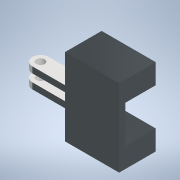
# Autodesk Inventor part: Tope_Carril
Saved by Autodesk Inventor 2022 (Build 260153000, 153)
## iProperties
Created: 2022-02-07
Part Number: Tope_Carril
Material: Generic
Document SubType Name: Modeling
Designer: katha
Density: 1 g/cm^3
Appearance: Default
Author: katha
Autodesk Inventor part; units mm, degrees
ref_plane "YZ Plane" through (0, 0, 0) normal (1, 0, 0) x (0, 1, 0)
ref_plane "XZ Plane" through (0, 0, 0) normal (0, 1, 0) x (-1, 0, 0)
ref_plane "XY Plane" through (0, 0, 0) normal (0, 0, 1) x (1, 0, 0)
sketch "Sketch1" plane through (0, 0, 0) normal (0, 0, 1) x (1, 0, 0)
  line L0 (0, 0) -> (20, 0) projected
  line L1 (20, 0) -> (20, 3.2) projected
  line L2 (0, 3.2) -> (20, 3.2) projected
  line L3 (0, 0) -> (0, 3.2) projected
  line L4 (20, -25) -> (0, -25) projected
  line L5 (0, -25) -> (0, -28.2) projected
  line L6 (20, -28.2) -> (0, -28.2) projected
  line L7 (20, -25) -> (20, -28.2) projected
  line L8 (3.2, -25) -> (3.2, 0) projected
  line L9 (0, -25) -> (0, 0) projected
  line L10 (-0.3, -0.3) -> (-0.3, 3.5)
  line L11 (-0.3, 3.5) -> (20.3, 3.5)
  line L12 (20.3, 3.5) -> (20.3, -0.3)
  line L13 (20.3, -24.7) -> (20.3, -28.5)
  line L14 (20.3, -28.5) -> (-0.3, -28.5)
  line L15 (-0.3, -28.5) -> (-0.3, -24.7)
  line L16 (3.5, -24.7) -> (3.5, -0.3)
  line L17 (-0.3, -0.3) -> (-0.3, -24.7)
  line L18 (20.3, -0.3) -> (3.5, -0.3)
  line L19 (3.5, -24.7) -> (20.3, -24.7)
  line L20 (6.5, -3.3) -> (6.5, -21.7)
  line L21 (6.5, -21.7) -> (23.3, -21.7)
  line L22 (23.3, -21.7) -> (23.3, -31.5)
  line L23 (23.3, -31.5) -> (-3.3, -31.5)
  line L24 (-3.3, -31.5) -> (-3.3, -24.7)
  line L25 (-3.3, -24.7) -> (-3.3, -0.3)
  line L26 (-3.3, -0.3) -> (-3.3, 6.5)
  line L27 (-3.3, 6.5) -> (23.3, 6.5)
  line L28 (23.3, 6.5) -> (23.3, -3.3)
  line L29 (23.3, -3.3) -> (6.5, -3.3)
  dimension "d2" = 0.3
  dimension "d3" = 0.3
  dimension "d4" = 0.3
  dimension "d5" = 24.4
  dimension "d6" = 3.8
  dimension "d7" = 3
  constraints: 40 end point, 3 equal length, 1 parallel, 13 other
  measures "d2" distance between parallel lines of L8 L16
  measures "d3" distance between parallel lines of L0 L18
  measures "d4" distance between parallel lines of L11 L2
  measures "d5" distance of L10.start L15.end
  measures "d6" distance of L10.start L10.end
  measures "d7" distance between parallel lines of L16 L20
extrude "Extrusion1" add sketch "Sketch1" against normal blind 15 contours L20 L21 L22 L23 L24 L25 L26 L27 L28 L29
sketch "Sketch4" plane through (0, 0, 0) normal (0, 0, 1) x (1, 0, 0)
  line L0 (23.3, -3.3) -> (23.3, 6.5) projected
  line L1 (23.3, 6.5) -> (-3.3, 6.5) projected
  line L2 (23.3, -3.3) -> (6.5, -3.3) projected
  line L3 (6.5, -3.3) -> (6.5, -21.7) projected
  line L4 (6.5, -21.7) -> (23.3, -21.7) projected
  line L5 (-3.3, -0.3) -> (-3.3, 6.5) projected
  line L6 (-3.3, -31.5) -> (23.3, -31.5) projected
  line L7 (23.3, -31.5) -> (23.3, -21.7) projected
  line L8 (23.3, -21.7) -> (6.5, -21.7) projected
  line L9 (23.3, 6.5) -> (23.3, -3.3) projected
  line L10 (23.3, -3.3) -> (23.3, 6.5)
  line L11 (-3.3, -31.5) -> (-3.3, 6.5) projected
  line L12 (23.3, 6.5) -> (-3.3, 6.5)
  line L13 (-3.3, 6.5) -> (-3.3, -31.5)
  line L14 (23.3, -31.5) -> (-3.3, -31.5) projected
  line L15 (-3.3, -31.5) -> (23.3, -31.5)
  line L16 (23.3, -21.7) -> (23.3, -31.5) projected
  line L17 (23.3, -31.5) -> (23.3, -21.7)
  line L18 (6.5, -3.3) -> (6.5, -21.7) projected
  line L19 (23.3, -3.3) -> (6.5, -3.3) projected
  line L20 (6.5, -3.3) -> (23.3, -3.3) projected
  line L21 (23.3, -3.3) -> (23.3, -21.7)
  point P0 (0, 0)
  constraints: 12 end point, 5 collinear, 1 perpendicular
extrude "Extrusion3" add sketch "Sketch4" along normal blind 3
sketch "Sketch5" plane through (6.5, -21.7, -15) normal (1, 0, 0) x (0, 0, -1)
  line L0 (0, 18.4) -> (0, 0) projected
  line L1 (-15, 18.4) -> (0, 18.4) projected
  line L2 (-15, 0) -> (0, 0) projected
  line L3 (-15, 0) -> (-15, 18.4) projected
  circle A0 centre (-6, 9.2) radius 2
  circle A1 centre (-6, 9.2) radius 4
  point P0 (-15, 21.7)
  dimension "d14" = 4
  dimension "d15" = 6
  dimension "d16" = 8
  dimension "d17" = 9.2
  constraints: 2 centre point, 1 coincident
  measures "d14" diameter of A0
  measures "d15" distance from line of L0 A0.centre
  measures "d16" diameter of A1
  measures "d17" distance from line of L1 A0.centre
extrude "Extrusion4" cut sketch "Sketch5" against normal blind 1 contours A1
extrude "Extrusion5" cut sketch "Sketch5" against normal blind 80 contours A0
sketch "Sketch16" plane through (-3.3, -31.5, -15) normal (-1, 0, 0) x (0, 0, 1)
  line L0 (18, 38) -> (18, 0) projected
  line L1 (0, 0) -> (18, 0) projected
  line L2 (18, 0) -> (18, 38) projected
  line L3 (18, 19) -> (0, 19) construction
  line L4 (0, 6.8) -> (0, 31.2) projected
  line L5 (18, 17.1) -> (18, 14.1)
  line L6 (18, 14.1) -> (9.94, 14.1)
  line L7 (9.94, 14.1) -> (9.94, 17.1)
  line L8 (9.94, 17.1) -> (18, 17.1)
  line L9 (18, 20.9) -> (18, 23.9)
  line L10 (18, 23.9) -> (9.94, 23.9)
  line L11 (9.94, 23.9) -> (9.94, 20.9)
  line L12 (9.94, 20.9) -> (18, 20.9)
  point P0 (15, 31.5)
  dimension "d41" = 3
  dimension "d42" = 1.9
  dimension "d43" = 8.06
  constraints: 18 end point, 4 symmetric about line, 2 midpoint, 2 parallel, 2 point on line, 1 perpendicular
  measures "d41" distance of L5.start L5.end
  measures "d42" distance between parallel lines of L8 L3
  measures "d43" distance between parallel lines of L7 L0
extrude "Extrusion8" add sketch "Sketch16" along normal blind 20.03
fillet "Fillet1" radius 4 4 edges at (-23.33, -15.9, 3) (-23.33, -9.1, 3) (-23.33, -9.1, -5.06) (-23.33, -15.9, -5.06)
sketch "Sketch17" plane through (-3.3, -17.4, -5.06) normal (0, -1, 0) x (1, 0, 0)
  arc A0 (-16.03, 8.06) -> (-20.03, 4.06) centre (-16.03, 4.06) ccw projected
  circle A1 centre (-16.03, 4.06) radius 2.03
  point P0 (3.3, 5.06)
  dimension "d47" = 4.06
  constraints: 1 centre point, 1 coincident
  measures "d47" diameter of A1
extrude "Extrusion9" cut sketch "Sketch17" against normal blind 20
body "Solid1"
